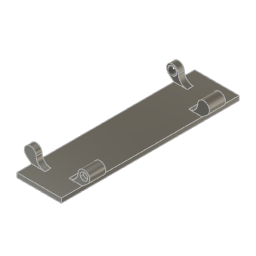
ogniwo-prototyp-v4-v1 (Autodesk Fusion 360 design; units mm, degrees)
Autodesk Fusion 360 part; units mm, degrees
sketch "Szkic1" plane through (0, 0, 0) normal (0, 0, 1) x (1, 0, 0)
  line L0 (0, 0) -> (15, 0)
  line L1 (15, 0) -> (15, 60)
  line L2 (15, 60) -> (0, 60)
  line L3 (0, 60) -> (0, 0)
  dimension "d1" = 15
  dimension "d2" = 60
  constraint horizontal L0
  constraint vertical L1
  constraint horizontal L2
  constraint vertical L3
  constraint coincident L0.start L3.end
  measures "d1" distance of L0.start L0.end
  measures "d2" distance of L0.start L2.end
extrude "Wyciągnięcie proste1" add sketch "Szkic1" along normal blind 1.5
sketch "Szkic2" plane through (0, 0, 0) normal (0, -1, 0) x (1, 0, 0)
  line L0 (0, 0) -> (15, 0)
  line L1 (15, 0) -> (15, 1.5)
  line L2 (15, 1.5) -> (0, 1.5)
  line L3 (0, 1.5) -> (0, 0)
  circle A0 centre (-0.5018, 4.5) radius 1.5
  circle A1 centre (-0.5018, 4.5) radius 2
  line L4 (0, 1.5) -> (-1.7711, 2.9544)
  line L5 (-0.5018, 4.5) -> (0.9124, 5.9142)
  line L6 (-0.5018, 4.5) -> (2, 4.5) construction
  line L7 (2, 4.5) -> (2, 4.5)
  line L8 (5, 1.5) -> (5, 1.5)
  line L9 (1.4982, 4.5) -> (1.4982, 4.5)
  line L10 (4.4982, 1.5) -> (4.4982, 1.5)
  arc A2 (1.4982, 4.5) -> (4.4982, 1.5) centre (4.4982, 4.5) ccw
  point P0 (2, 1.5)
  point P1 (1.4982, 1.5)
  dimension "d5" = 45
  dimension "d6" = 3
  dimension "d18" = 3
  dimension "d19" = 3
  constraint coincident L2.end L3.start
  constraint concentric A0 A1
  constraint coincident A1 L4.end
  constraint tangent A1 L4
  constraint horizontal L6
  constraint coincident A0.centre A1.centre
  constraint coincident A1 L5.end
  constraint coincident L2 P0
  constraint coincident P0 L7
  constraint coincident P0 L8
  constraint coincident A1 L9.start
  constraint coincident L6 L9.start
  constraint coincident L2 P1
  constraint coincident P1 L9
  constraint coincident P1 L10
  measures "d5" angle of L5 L6
  measures "d6" distance of P0 L8.start
  measures "d18" distance of P1 L10.start
  measures "d19" radius of A2
extrude "Wyciągnięcie proste2" add sketch "Szkic2" against normal blind 2 from surface at -5 contours L2 A1 L4 A2 | A1 | A0
sketch "Szkic3" plane through (0, 7, 0) normal (0, 1, 0) x (-1, 0, 0)
  arc A0 (1.7711, 2.9544) -> (-1.4982, 4.5) centre (0.5018, 4.5) ccw
  line L0 (-4.4982, 1.5) -> (0, 1.5)
  line L1 (0, 1.5) -> (1.7711, 2.9544)
  circle A1 centre (0.5018, 4.5) radius 1.5
  line L2 (0.5018, 4.5) -> (2.0018, 4.5)
  arc A2 (-4.4982, 1.5) -> (-1.4982, 4.5) centre (-4.4982, 4.5) ccw
  dimension "d11" = 3
  constraint concentric A0 A1
  constraint coincident A0.centre A1.centre
  constraint coincident A1 L2.end
  constraint horizontal L2
  measures "d11" diameter of A1
sketch "Szkic5" plane through (0, 0, 4.5) normal (0, 0, -1) x (1, 0, 0)
  line L0 (-0.5018, -7) -> (-2.0018, -7)
  line L1 (-2.0018, -7) -> (-2.0018, -8)
  line L2 (-2.0018, -8) -> (-0.5018, -8)
  line L3 (-0.5018, -8) -> (-0.5018, -7)
  line L4 (-2.0018, -7) -> (1, -7)
  arc A0 (-2.0018, -7) -> (1, -7) centre (-0.5009, -6.3736) ccw
  constraint coincident L0.end L1.start
  constraint perpendicular L3 L4
  constraint coincident L2.end A0
revolve "Obrót2" add sketch "Szkic5" angle 360 about axis through (-0.5018, 8, 4.5) along (0, -1, 0) contours L0 L3 L4 A0
sketch "Szkic6" plane through (0, 0, 0) normal (0, -1, 0) x (1, 0, 0)
  circle A0 centre (15.5, 4.5) radius 1.3
  circle A1 centre (15.5, 4.5) radius 2
  line L0 (15, 1.5) -> (16.77, 2.955)
  line L1 (13.5, 4.5) -> (13.5, 4.5)
  line L2 (10.5, 1.5) -> (10, 1.5)
  line L3 (13.5, 1.5) -> (15, 1.5)
  arc A2 (10.5, 1.5) -> (13.5, 4.5) centre (10.5, 4.5) ccw
  line L4 (10, 1.5) -> (10.1, 1.5)
  line L5 (13.5, 1.5) -> (10.25, 1.5)
  dimension "d26" = 2.6
  dimension "d27" = 3
  constraint coincident A1 L0.end
  constraint tangent A1 L0
  constraint coincident A1 L1.start
  constraint coincident L3.start L1
  constraint coincident L3.start L2
  constraint tangent L2 A2
  constraint coincident L2 L4.end
  constraint midpoint L2 L5.end
  constraint parallel L2 L5
  measures "d26" diameter of A0
  measures "d27" radius of A2
extrude "Wyciągnięcie proste7" add sketch "Szkic6" against normal blind 5 from surface at -7.5 contours A0 | A1 | A1 L0 L3 A2 L5
sketch "Szkic7" plane through (0, 7.5, 0) normal (0, -1, 0) x (1, 0, 0)
  line L0 (15, 1.5) -> (16.77, 2.955)
  arc A0 (16.77, 2.955) -> (13.5, 4.5) centre (15.5, 4.5) ccw
  arc A1 (10.5, 1.5) -> (13.5, 4.5) centre (10.5, 4.5) ccw
  line L1 (10.5, 1.5) -> (15, 1.5)
  circle A2 centre (15.5, 4.5) radius 1.25
  dimension "d31" = 2.5
  constraint concentric A0 A2
  measures "d31" diameter of A2
extrude "Wyciągnięcie proste8" cut sketch "Szkic7" against normal blind 0.6 contours A2
extrude "Wyciągnięcie proste9" add sketch "Szkic2" along normal blind 2 from surface at -55 contours L2 A1 L4 A2 | A1 | A0
sketch "Szkic8" plane through (0, 53, 0) normal (0, -1, 0) x (1, 0, 0)
  arc A0 (1.4982, 4.5) -> (-1.7711, 2.9544) centre (-0.5018, 4.5) ccw
  line L0 (-1.7711, 2.9544) -> (0, 1.5)
  line L1 (0, 1.5) -> (4.4982, 1.5)
  arc A1 (1.4982, 4.5) -> (4.4982, 1.5) centre (4.4982, 4.5) ccw
  circle A2 centre (-0.5018, 4.5) radius 1.5
  line L2 (-0.5018, 4.5) -> (-2.0018, 4.5)
  dimension "d37" = 3
  constraint concentric A0 A2
  constraint coincident A0.centre A2.centre
  constraint coincident A2 L2.end
  constraint horizontal L2
  measures "d37" diameter of A2
sketch "Szkic9" plane through (0, 0, 4.5) normal (0, 0, 1) x (-1, 0, 0)
  line L0 (0.5018, -53) -> (2.0018, -53)
  line L1 (2.0018, -53) -> (2.0018, -52)
  line L2 (2.0018, -52) -> (0.5018, -52)
  line L3 (0.5018, -52) -> (0.5018, -53)
  line L4 (2.0018, -53) -> (-0.9982, -53)
  arc A0 (2.0018, -53) -> (-0.9982, -53) centre (0.5018, -53.625) ccw
  dimension "d40" = 3
  constraint coincident L0.end L1.start
  constraint perpendicular L1 L4
  constraint coincident L2.end A0
  measures "d40" distance of L0.end L4.end
revolve "Obrót3" add sketch "Szkic9" angle 360 about axis through (-0.5018, 52, 4.5) along (0, 1, 0) contours L0 L3 L4 A0
extrude "Wyciągnięcie proste11" add sketch "Szkic6" along normal blind 5 from surface at -52.5 contours A0 | A1 | A1 L0 L3 A2 L5
sketch "Szkic10" plane through (0, 52.5, 0) normal (0, 1, 0) x (-1, 0, 0)
  line L0 (-16.77, 2.955) -> (-15, 1.5)
  line L1 (-15, 1.5) -> (-10.5, 1.5)
  arc A0 (-13.5, 4.5) -> (-10.5, 1.5) centre (-10.5, 4.5) ccw
  arc A1 (-13.5, 4.5) -> (-16.77, 2.955) centre (-15.5, 4.5) ccw
  circle A2 centre (-15.5, 4.5) radius 1.25
  dimension "d45" = 2.5
  constraint concentric A1 A2
  measures "d45" diameter of A2
extrude "Wyciągnięcie proste12" cut sketch "Szkic10" against normal blind 0.6 contours A2
extrude "Wyciągnięcie proste13" add 1 faces at (14.4583, 7.5, 2.1392) along direction (0, -1, 0) blind 0.4
extrude "Wyciągnięcie proste14" add sketch "Szkic10" along normal blind 0.4
